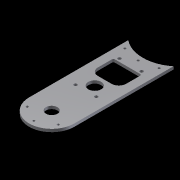
# Autodesk Inventor part: JointC2cover_2nd
Saved by Autodesk Inventor 2011 SP1 (Build 150282100, 282)
## iProperties
Created: 2013-02-08
Part Number: JointC2cover_2nd
Document SubType Name: Modeling
Designer: arihon
Density: 1 g/cm^3
Author: arihon
Autodesk Inventor part; units mm, degrees
ref_plane "YZ Plane" through (0, 0, 0) normal (1, 0, 0) x (0, 1, 0)
ref_plane "XZ Plane" through (0, 0, 0) normal (0, 1, 0) x (-1, 0, 0)
ref_plane "XY Plane" through (0, 0, 0) normal (0, 0, 1) x (1, 0, 0)
sketch "スケッチ1" plane through (0, 0, 0) normal (0, 0, 1) x (1, 0, 0)
  circle A0 centre (-10.8253, -50.5) radius 0.7835
  circle A1 centre (0, -56.75) radius 0.7835
  circle A2 centre (10.8253, -50.5) radius 0.7835
  circle A3 centre (11.9284, 18.6695) radius 0.7835
  circle A4 centre (0, 16.025) radius 0.7835
  circle A5 centre (-11.9284, 18.6695) radius 0.7835
  line L0 (-9.85, -18.05) -> (-9.85, -7.35)
  arc A6 (-6.8, 12.8) -> (-9.85, 9.75) centre (-6.8, 9.75) ccw
  line L1 (-6.8, 12.8) -> (6.8, 12.8)
  arc A7 (9.85, 9.75) -> (6.8, 12.8) centre (6.8, 9.75) ccw
  line L2 (9.85, 9.75) -> (9.85, 8.57)
  arc A8 (4.8, -23.1) -> (9.85, -18.05) centre (4.8, -18.05) ccw
  line L3 (4.8, -23.1) -> (-4.8, -23.1)
  arc A9 (-9.85, -18.05) -> (-4.8, -23.1) centre (-4.8, -18.05) ccw
  circle A10 centre (0, -44.25) radius 4
  arc A11 (-15.75, 24.8351) -> (15.75, 24.8351) centre (0, 44.25) ccw
  line L4 (-15.75, -44.25) -> (-15.75, 24.8351)
  arc A12 (-15.75, -44.25) -> (15.75, -44.25) centre (0, -44.25) ccw
  line L5 (15.75, 24.8351) -> (15.75, -44.25)
  line L6 (-9.85, 8.57) -> (9.85, 8.57)
  line L7 (9.85, 8.57) -> (9.85, -7.35)
  line L8 (9.85, -7.35) -> (-9.85, -7.35)
  line L9 (-9.85, -7.35) -> (-9.85, 8.57)
  line L10 (9.85, 8.57) -> (9.85, -7.35)
  line L11 (-9.85, 8.57) -> (-9.85, 9.75)
  line L12 (-9.85, -7.35) -> (-9.85, 8.57)
  line L13 (9.85, -7.35) -> (9.85, -18.05)
  point P0 (0, 0)
  point P1 (0, 0)
  dimension "d3" = 4.23
  dimension "d4" = 15.75
  constraints: 28 end point, 13 centre point, 12 point on circle, 2 parallel, 1 horizontal, 1 perpendicular, 1 point on line
  measures "d3" distance between parallel lines of L6 L1
  measures "d4" distance between parallel lines of L3 L8
extrude "押し出し2" add sketch "スケッチ1" along normal blind 2 contours L0 L8 L13 A8 L3 A9 | L11 A6 L1 A7 L2 L6 | A11 L5 A12 L4
sketch "スケッチ2" plane through (0, 0, 2) normal (0, 0, 1) x (1, 0, 0)
  line L0 (9.85, -7.35) -> (-9.85, -7.35) projected
  line L1 (15.75, 24.8351) -> (15.75, -44.25) projected
  line L2 (-15.75, -44.25) -> (-15.75, 24.8351) projected
  line L3 (0, 18.6695) -> (0, -60)
  point P0 (0, 0)
  point P1 (0, 0)
  point P2 (-7.7, 10.65)
  point P3 (-7.2, -20.45)
  point P4 (7.2, -20.45)
  point P5 (7.7, 10.65)
  point P6 (0, -14.25)
  dimension "d10" = 31.1
  dimension "d11" = 31.1
  dimension "d12" = 15.4
  dimension "d13" = 14.4
  dimension "d14" = 15.4
  dimension "d15" = 31.5
  dimension "d16" = 14.4
  dimension "d26" = 6.9
  dimension "d27" = 6.2
  dimension "d28" = 6.2
  constraints: 2 end point, 1 parallel, 1 point on line
  measures "d10" vertical distance of point (7.2, -20.45) point (7.7, 10.65)
  measures "d11" vertical distance of point (-7.2, -20.45) point (-7.7, 10.65)
  measures "d12" distance of point (7.7, 10.65) point (-7.7, 10.65)
  measures "d13" distance of point (-7.2, -20.45) point (7.2, -20.45)
  measures "d14" diameter of point (-7.7, 10.65) L3
  measures "d15" diameter of L1 L3
  measures "d16" diameter of point (7.2, -20.45) L3
  measures "d26" distance from line of point (0, -14.25) L0
  measures "d27" vertical distance of point (7.2, -20.45) point (0, -14.25)
  measures "d28" vertical distance of point (-7.2, -20.45) point (0, -14.25)
hole "Hole2" at (7.7, 10.65, 2) at (7.2, -20.45, 2) at (-7.2, -20.45, 2) at (-7.7, 10.65, 2) at (0, -14.25, 2) direction (0, 0, -1) diameter 2.2 depth 8 tip angle 118
sketch "スケッチ4" plane through (0, 0, 2) normal (0, 0, 1) x (1, 0, 0)
  point P0 (0, 0)
  point P1 (0, -14.25)
hole "Hole3" at (0, -14.25, 2) direction (0, 0, -1) diameter 9 depth 8 tip angle 118
fillet "フィレット3" radius 1.05 2 edges at (-9.85, 8.57, 1) (9.85, 8.57, 1)
fillet "フィレット4" radius 5.05 2 edges at (-9.85, -7.35, 1) (9.85, -7.35, 1)
sketch "スケッチ6" plane through (0, 0, 0) normal (0, 0, -1) x (-1, 0, 0)
  circle A0 centre (-10.8253, -50.5) radius 0.7835 projected
  circle A1 centre (0, -56.75) radius 0.7835 projected
  circle A2 centre (10.8253, -50.5) radius 0.7835 projected
  circle A3 centre (0, -44.25) radius 10.5
  circle A4 centre (0, -44.25) radius 14.5
  point P0 (0, 0)
  dimension "d50" = 21
  dimension "d51" = 29
  constraints: 2 centre point
  measures "d50" diameter of A3
  measures "d51" diameter of A4
extrude "押し出し4" cut sketch "スケッチ6" against normal blind 1
equation "\"d11\" = d10"
equation "\"d14\" = d12"
equation "\"d16\" = d13"
